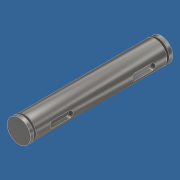
# Autodesk Inventor part: AxeVerticalManivelle
Saved by Autodesk Inventor 2018 (Build 220112000, 112)
## iProperties
Created: 2022-03-25
Part Number: AxeVerticalManivelle
Material: Stainless Steel
Document SubType Name: Modeling
Designer: Nathann
Density: 8 g/cm^3
Appearance: Semi-Polished
Mass: 35.4464 g
Surface Area: 23.8023 cm^2
Volume: 4.4308 cm^3
Author: Nathann
Autodesk Inventor part; units mm, degrees
ref_plane "XZ Plane" through (0, 0, 0) normal (0, 1, 0) x (-1, 0, 0)
ref_plane "XY Plane" through (0, 0, 0) normal (0, 0, 1) x (1, 0, 0)
sketch "Sketch1" plane through (0, 0, 0) normal (0, 1, 0) x (-1, 0, 0)
  arc A0 (4.7697, 1.5) -> (4.7697, -1.5) centre (0, 0) ccw
  circle A1 centre (0, 0) radius 5
  dimension "d0" = 10
  constraints: 2 coincident, 2 point on circle, 1 centre point, 3 other
  measures "d0" diameter of A0
extrude "Extrusion1" add sketch "Sketch1" along normal blind 58.3
sketch "Sketch2" plane through (0, 0, 0) normal (0, -1, 0) x (1, 0, 0)
  arc A0 (-4.7697, -1.5) -> (-4.7697, 1.5) centre (0, 0) ccw projected
  line L0 (-3.2, 1.5) -> (-4.7697, 1.5) projected
  line L1 (-3.2, -1.5) -> (-3.2, 1.5) projected
  line L2 (-4.7697, -1.5) -> (-3.2, -1.5) projected
  circle A1 centre (0, 0) radius 5
  constraints: 1 centre point, 1 coincident, 1 concentric
extrude "Extrusion2" add sketch "Sketch2" along normal blind 3
sketch "Sketch3" plane through (0, 0, 0) normal (0, 0, 1) x (1, 0, 0)
  line L0 (7.5, -1.5) -> (3.5, -1.5)
  line L1 (3.5, -1.5) -> (3.5, -0.56)
  line L2 (3.5, -0.56) -> (7.5, -0.56)
  line L3 (7.5, -0.56) -> (7.5, -1.5)
  line L4 (-4.7697, -3) -> (5, -3) projected
  line L5 (5, -3) -> (5, 58.3) projected
  line L6 (0, -15.26) -> (0, 70.56) projected
  line L7 (5, -3) -> (5, 58.3) projected
  line L8 (5, 27.65) -> (17.8962, 27.65)
  line L9 (7.5, 56.8) -> (3.5, 56.8)
  line L10 (3.5, 56.8) -> (3.5, 55.86)
  line L11 (3.5, 55.86) -> (7.5, 55.86)
  line L12 (7.5, 55.86) -> (7.5, 56.8)
  point P0 (0, 0)
  point P1 (0, 55.3)
  dimension "d10" = 0.94
  dimension "d11" = 4
  dimension "d12" = 1.5
  dimension "d21" = 1.5
  constraints: 18 end point, 8 symmetric about line, 2 horizontal, 2 parallel, 1 midpoint, 1 perpendicular
  measures "d10" distance of L2.end L0.start
  measures "d11" distance of L0.start L0.end
  measures "d12" distance between parallel lines of L5 L1
  measures "d21" distance between parallel lines of L4 L0
revolve "Revolution1" cut sketch "Sketch3" angle 360 about axis through (0, -10, 0) along (0, 1, 0)
ref_plane "Work Plane1" through (5, 0, 0) normal (1, 0, 0) x (0, 1, 0)
sketch "Sketch6" plane through (5, 0, 0) normal (1, 0, 0) x (0, 1, 0)
  line L0 (6.94, 1.5) -> (13.94, 1.5)
  line L1 (13.94, 1.5) -> (13.94, -1.5)
  line L2 (13.94, -1.5) -> (6.94, -1.5)
  line L3 (6.94, -1.5) -> (6.94, 1.5)
  circle A0 centre (6.94, 0) radius 1.5
  circle A1 centre (13.94, 0) radius 1.5
  line L4 (-0.56, 5) -> (55.86, 5) projected
  line L5 (-0.56, -5) -> (55.86, -5) projected
  line L6 (42.36, 1.5) -> (49.36, 1.5)
  line L7 (49.36, 1.5) -> (49.36, -1.5)
  line L8 (49.36, -1.5) -> (42.36, -1.5)
  line L9 (42.36, -1.5) -> (42.36, 1.5)
  circle A2 centre (42.36, 0) radius 1.5
  circle A3 centre (49.36, 0) radius 1.5
  line L10 (-3, 5) -> (-3, -5) projected
  line L11 (58.3, -5) -> (58.3, 5) projected
  line L12 (-0.56, -5) -> (-0.56, 5) projected
  line L13 (55.86, 5) -> (55.86, -5) projected
  point P0 (0, 0)
  dimension "d26" = 3
  dimension "d22" = 3
  dimension "d23" = 3.5
  dimension "d24" = 7
  dimension "d25" = 7
  dimension "d27" = 3.5
  dimension "d33" = 7.5
  dimension "d34" = 6.5
  constraints: 16 end point, 4 midpoint, 4 parallel, 4 vertical alignment, 2 horizontal, 2 perpendicular, 8 other
  measures "d22" distance between parallel lines of L2 L0
  measures "d23" distance between parallel lines of L4 L0
  measures "d24" distance of point (13.94, 0) point (6.94, 0)
  measures "d25" distance of point (49.36, 0) point (42.36, 0)
  measures "d27" distance between parallel lines of L4 L6
  measures "d33" distance from line of point (6.94, 0) L12
  measures "d34" distance from line of point (49.36, 0) L13
extrude "Extrusion4" cut sketch "Sketch6" against normal blind 1.8 contours A0 L3 | L0 A1 L2 A0 | L3 A0 | A1 L1 | L1 A1 | A2 L9 | L6 A3 L8 A2 | L9 A2 | A3 L7 | L7 A3
body "Solid1"
